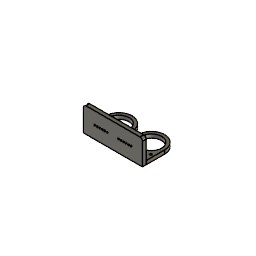
sensorHolder (Autodesk Fusion 360 design; units mm, degrees)
part number: 2026-05-30-15-33-03-578
Autodesk Fusion 360 part; units mm, degrees
sketch "Sketch1" plane through (0, 14.27, 0) normal (0, 1, 0) x (-1, 0, 0)
  circle A0 centre (-1.3, -5.9) radius 0.5 construction
  circle A1 centre (2.7, -5.9) radius 0.5 construction
  circle A2 centre (6.7, -5.9) radius 0.5 construction
  circle A3 centre (8.7, -5.9) radius 0.5 construction
  circle A4 centre (4.7, -5.9) radius 0.5 construction
  circle A5 centre (0.7, -5.9) radius 0.5 construction
  circle A6 centre (-10.5, -5.9) radius 0.5 construction
  circle A7 centre (-14.5, -5.9) radius 0.5 construction
  circle A8 centre (-18.5, -5.9) radius 0.5 construction
  circle A9 centre (-20.5, -5.9) radius 0.5 construction
  circle A10 centre (-16.5, -5.9) radius 0.5 construction
  circle A11 centre (-12.5, -5.9) radius 0.5 construction
  circle A12 centre (-5.9, -5.9) radius 2.425 construction
  arc A13 (-8.0333, -8.775) -> (-3.7667, -8.775) centre (-5.9, -5.9) ccw construction
  line L0 (-3.7667, -8.775) -> (8.2462, -7.8947) construction
  arc A14 (8.2462, -7.8947) -> (8.2462, -3.9053) centre (8.1, -5.9) ccw construction
  line L1 (8.2462, -3.9053) -> (-3.7667, -3.025) construction
  arc A15 (-3.7667, -3.025) -> (-8.0333, -3.025) centre (-5.9, -5.9) ccw construction
  line L2 (-8.0333, -3.025) -> (-20.0462, -3.9053) construction
  arc A16 (-20.0462, -3.9053) -> (-20.0462, -7.8947) centre (-19.9, -5.9) ccw construction
  line L3 (-20.0462, -7.8947) -> (-8.0333, -8.775) construction
  line L4 (17.92, -15.9) -> (-29.72, -15.9)
  line L5 (-29.72, -15.9) -> (-29.72, 4.1)
  line L6 (-29.72, 4.1) -> (17.92, 4.1)
  line L7 (17.92, 4.1) -> (17.92, -15.9)
  line L8 (17.92, -15.9) -> (-29.72, 4.1) construction
  line L9 (-29.72, -15.9) -> (17.92, 4.1) construction
  circle A17 centre (8.7, -5.9) radius 0.65
  circle A18 centre (-20.5, -5.9) radius 0.65
  circle A19 centre (6.7, -5.9) radius 0.65
  circle A20 centre (4.7, -5.9) radius 0.65
  circle A21 centre (2.7, -5.9) radius 0.65
  circle A22 centre (0.7, -5.9) radius 0.65
  circle A23 centre (-1.3, -5.9) radius 0.65
  circle A24 centre (-18.5, -5.9) radius 0.65
  circle A25 centre (-16.5, -5.9) radius 0.65
  circle A26 centre (-14.5, -5.9) radius 0.65
  circle A27 centre (-12.5, -5.9) radius 0.65
  circle A28 centre (-10.5, -5.9) radius 0.65
  point P0 (-5.9, -5.9)
  dimension "d1" = 20
  dimension "d2" = 47.64
  dimension "d3" = 1.3
  dimension "d4" = 1.3
  dimension "d30" = 1.3
  dimension "d31" = 1.3
  dimension "d32" = 1.3
  dimension "d33" = 1.3
  dimension "d34" = 1.3
  dimension "d35" = 1.3
  dimension "d36" = 1.3
  dimension "d37" = 1.3
  dimension "d38" = 1.3
  dimension "d39" = 1.3
  constraint horizontal L4
  constraint perpendicular L4 L5
  constraint parallel L4 L6
  constraint parallel L5 L7
  constraint coincident L8 P0
  constraint coincident L9 P0
  constraint coincident P0 A12.centre
  constraint concentric A3 A17
  constraint concentric A9 A18
  constraint concentric A2 A19
  constraint concentric A4 A20
  constraint concentric A1 A21
  constraint concentric A5 A22
  constraint concentric A0 A23
  constraint concentric A8 A24
  constraint concentric A10 A25
  constraint concentric A7 A26
  constraint concentric A11 A27
  constraint concentric A6 A28
  measures "d1" distance of L4.start L6.end
  measures "d2" distance of L5.end L6.end
  measures "d3" diameter of A17
  measures "d4" diameter of A18
  measures "d30" diameter of A19
  measures "d31" diameter of A20
  measures "d32" diameter of A21
  measures "d33" diameter of A22
  measures "d34" diameter of A23
  measures "d35" diameter of A24
  measures "d36" diameter of A25
  measures "d37" diameter of A26
  measures "d38" diameter of A27
  measures "d39" diameter of A28
extrude "Extrude1" add sketch "Sketch1" along normal blind 3 makes body 1
sketch "Sketch3" plane through (0, 0, -15.9) normal (0, 0, -1) x (1, 0, 0)
  line L0 (29.72, -15.22) -> (-17.92, -15.22)
  line L1 (-17.92, -15.22) -> (-17.92, -18.22)
  line L2 (-17.92, -18.22) -> (29.72, -18.22)
  line L3 (29.72, -18.22) -> (29.72, -15.22)
  circle A0 centre (-15.525, -23.52) radius 0.75
  circle A1 centre (27.325, -23.52) radius 0.75
  line L4 (29.72, -18.22) -> (-17.92, -18.22)
  line L5 (-17.92, -18.22) -> (-17.92, -48.22)
  line L6 (-17.92, -48.22) -> (29.72, -48.22)
  line L7 (29.72, -48.22) -> (29.72, -18.22)
  circle A2 centre (-15.525, -23.52) radius 0.85
  circle A3 centre (27.325, -23.52) radius 0.85
  circle A4 centre (-7.22, -32.22) radius 8
  circle A5 centre (19.02, -32.22) radius 8
  circle A6 centre (19.02, -32.22) radius 8.2
  circle A7 centre (-7.22, -32.22) radius 8.2
  line L8 (19.02, -32.22) -> (-7.22, -32.22) construction
  arc A8 (9.1, -27.0844) -> (11.3, -24.8844) centre (9.1, -24.8844) ccw
  line L9 (2.7, -27.0844) -> (9.1, -27.0844)
  arc A9 (0.5, -24.8844) -> (2.7, -27.0844) centre (2.7, -24.8844) ccw
  arc A10 (2.7, -22.5844) -> (0.5, -24.7844) centre (2.7, -24.7844) ccw
  line L10 (9.1, -22.5844) -> (2.7, -22.5844)
  arc A11 (11.3, -24.7844) -> (9.1, -22.5844) centre (9.1, -24.7844) ccw
  line L11 (9.1, -27.2844) -> (2.7, -27.2844)
  line L12 (2.7, -22.3844) -> (9.1, -22.3844)
  arc A12 (2.7, -22.3844) -> (0.3005, -24.8344) centre (2.7, -24.7844) ccw
  arc A13 (0.3005, -24.8344) -> (2.7, -27.2844) centre (2.7, -24.8844) ccw
  arc A14 (9.1, -27.2844) -> (11.4995, -24.8344) centre (9.1, -24.8844) ccw
  arc A15 (11.4995, -24.8344) -> (9.1, -22.3844) centre (9.1, -24.7844) ccw
  arc A16 (0.2005, -24.8344) -> (2.7, -27.3844) centre (2.7, -24.8844) ccw
  line L13 (9.1, -27.3844) -> (2.7, -27.3844)
  arc A17 (9.1, -27.3844) -> (11.5995, -24.8344) centre (9.1, -24.8844) ccw
  arc A18 (11.5995, -24.8344) -> (9.1, -22.2844) centre (9.1, -24.7844) ccw
  line L14 (2.7, -22.2844) -> (9.1, -22.2844)
  arc A19 (2.7, -22.2844) -> (0.2005, -24.8344) centre (2.7, -24.7844) ccw
  dimension "d7" = 1.7
  dimension "d8" = 1.7
  dimension "d11" = 30
  dimension "d12" = 16.4
  dimension "d13" = 16.4
  dimension "d42" = -0.1
  constraint horizontal L4
  constraint vertical L5
  constraint horizontal L6
  constraint vertical L7
  constraint coincident L2.end L3.start
  constraint coincident L1.end L2.start
  constraint concentric A0 A2
  constraint concentric A1 A3
  constraint concentric A5 A6
  constraint concentric A4 A7
  constraint coincident A5.centre A6.centre
  constraint concentric A9 A13
  constraint tangent L11 A13
  constraint concentric A10 A12
  constraint tangent L12 A12
  constraint concentric A8 A14
  constraint tangent L11 A14
  constraint concentric A11 A15
  constraint tangent L12 A15
  measures "d7" diameter of A2
  measures "d8" diameter of A3
  measures "d11" distance of L2.end L6.end
  measures "d12" diameter of A7
  measures "d13" diameter of A6
extrude "Extrude2" add sketch "Sketch3" against normal blind 3 contours L2 L4 L5 L6 L7 | A16 L13 A17 A18 L14 A19 bodies 1 makes body 2
sketch "Sketch5" plane through (-17.92, 0, 0) normal (-1, 0, 0) x (0, -1, 0)
  line L0 (-14.27, -15.9) -> (-14.27, 4.1)
  line L1 (-14.27, 4.1) -> (-17.27, 4.1)
  line L2 (-17.27, 4.1) -> (-17.27, -15.9)
  line L3 (-17.27, -15.9) -> (-14.27, -15.9)
  line L4 (-17.27, -15.9) -> (-17.6705, -12.9269)
  line L5 (-17.27, -15.9) -> (-20.27, -15.9)
  line L6 (-20.27, -15.9) -> (-17.6705, -12.9269)
  dimension "d16" = 3
  dimension "d17" = 3
  constraint coincident L2.end L3.start
  constraint perpendicular L2 L5
  measures "d16" distance of L2.end L4.end
  measures "d17" distance of L2.end L5.end
extrude "Extrude3" add sketch "Sketch5" against normal up to surface (47.64 mm away) contours L4 L5 L6 bodies 1 2
sketch "Sketch6" plane through (0, 0, -15.9) normal (0, 0, -1) x (1, 0, 0)
  circle A0 centre (27.325, -23.52) radius 0.85
  circle A1 centre (-7.22, -32.22) radius 8.2
  circle A2 centre (-15.525, -23.52) radius 0.85
  circle A3 centre (19.02, -32.22) radius 8.2
  line L0 (29.72, -15.22) -> (-17.92, -15.22)
  line L1 (-17.92, -15.22) -> (-17.92, -48.22)
  line L2 (-17.92, -48.22) -> (29.72, -48.22)
  line L3 (29.72, -48.22) -> (29.72, -15.22)
  circle A4 centre (19.02, -32.22) radius 8
  circle A5 centre (-7.22, -32.22) radius 8
  circle A6 centre (19.02, -32.22) radius 10.7
  circle A7 centre (-7.22, -32.22) radius 10.7
  line L4 (19.02, -32.22) -> (-7.22, -32.22) construction
  line L5 (8.32, -32.22) -> (3.48, -32.22)
  line L6 (29.72, -48.22) -> (-17.92, -48.22)
  arc A8 (9.1, -27.2844) -> (11.4995, -24.8344) centre (9.1, -24.8844) ccw
  line L7 (9.1, -27.2844) -> (2.7, -27.2844)
  arc A9 (0.3005, -24.8344) -> (2.7, -27.2844) centre (2.7, -24.8844) ccw
  arc A10 (2.7, -22.3844) -> (0.3005, -24.8344) centre (2.7, -24.7844) ccw
  line L8 (2.7, -22.3844) -> (9.1, -22.3844)
  arc A11 (11.4995, -24.8344) -> (9.1, -22.3844) centre (9.1, -24.7844) ccw
  dimension "d22" = 21.4
  dimension "d23" = 21.4
  constraint concentric A4 A6
  constraint concentric A5 A7
  constraint coincident A3.centre A4.centre
  constraint coincident A1.centre A5.centre
  constraint coincident A6 L5.start
  constraint coincident L4 L5.start
  constraint coincident L4 L5.end
  constraint coincident A7 L5.end
  constraint coincident L2.end L3.start
  constraint coincident L1.end L2.start
  measures "d22" diameter of A6
  measures "d23" diameter of A7
extrude "Extrude4" cut sketch "Sketch6" against normal blind 3 contours L1 L2 L3 A6 A7 L5 L6 bodies 1
fillet "Fillet1" radius 2 1 edges at (-17.92, 15.77, 4.1) on bodies 1
fillet "Fillet2" radius 2 1 edges at (29.72, 15.77, 4.1) on bodies 1
